Game Controller PCB v4 (Autodesk Fusion 360 design; units mm, degrees)
Autodesk Fusion 360 part; units mm, degrees
sketch "Sketch5" plane through (0, 0, 0) normal (0, 0, 1) x (1, 0, 0) in component "case"
  line L0 (-57.6, 75) -> (57.6, 75)
  line L1 (57.6, 75) -> (97.6, 5.718)
  line L2 (97.6, 5.718) -> (78.1684, -17.1384)
  line L3 (78.1684, -17.1384) -> (42.026, 0)
  line L4 (42.026, 0) -> (-42.026, 0)
  line L5 (-42.026, 0) -> (-78.1684, -17.1384)
  line L6 (-78.1684, -17.1384) -> (-97.6, 5.718)
  line L7 (-97.6, 5.718) -> (-57.6, 75)
  line L8 (0, 0) -> (0, 150) construction
  dimension "d31" = 57.6
  dimension "d32" = 80
  dimension "d34" = 80
  dimension "d35" = 120
  dimension "d36" = 120
  dimension "d37" = 30
  dimension "d38" = 40
  dimension "d39" = 30
  dimension "d40" = 40
  dimension "d41" = 105
  dimension "d42" = 105
  dimension "d43" = 75
  dimension "d44" = 57.6
  constraint horizontal L0
  constraint parallel L0 L4
  constraint midpoint L8.start L4
  constraint coincident L8.start origin
  constraint perpendicular L0 L8
  constraint midpoint L0 L8
  measures "d31" distance of L0.end L8
  measures "d32" distance of L0.start L6.end
  measures "d34" distance of L0.end L1.end
  measures "d35" angle of L0 L7
  measures "d36" angle of L0 L1
  measures "d37" distance of L1.end L2.end
  measures "d38" distance of L2.end L3.end
  measures "d39" distance of L5.end L6.end
  measures "d40" distance of L4.end L5.end
  measures "d41" angle of L2 L3
  measures "d42" angle of L5 L6
  measures "d43" distance of L0 L4
  measures "d44" distance of L0.start L8
extrude "Extrude1" add sketch "Sketch5" along normal blind 20 in component "case"
fillet "Fillet1" radius 10 8 edges at (42.026, 0, 10) (-42.026, 0, 10) (-78.1684, -17.1384, 10) (78.1684, -17.1384, 10) (97.6, 5.718, 10) (57.6, 75, 10) (-57.6, 75, 10) (-97.6, 5.718, 10) in component "case"
shell "Shell1" thickness 3 removed faces 1 at (-13.2584, 50, 20) in component "case"
sketch "Sketch7" plane through (0, 0, 3) normal (0, 0, 1) x (-1, 0, 0) in component "case"
  arc A0 (91.4768, -10.3237) -> (90.7478, -2.2897) centre (85.4146, -6.8237) ccw
  line L0 (90.7478, -2.2897) -> (80.8529, 9.3491)
  arc A1 (80.8529, 9.3491) -> (72.5205, 11.14) centre (75.5198, 4.8151) ccw
  line L1 (72.5205, 11.14) -> (45.3451, -1.7463)
  arc A2 (39.7752, -3) -> (45.3451, -1.7463) centre (39.7752, 10) ccw
  line L2 (39.7752, -3) -> (-39.7752, -3)
  arc A3 (-45.3451, -1.7463) -> (-39.7752, -3) centre (-39.7752, 10) ccw
  line L3 (-45.3451, -1.7463) -> (-72.5205, 11.14)
  arc A4 (-72.5205, 11.14) -> (-80.8529, 9.3491) centre (-75.5198, 4.8151) ccw
  line L4 (-80.8529, 9.3491) -> (-90.7478, -2.2897)
  arc A5 (-90.7478, -2.2897) -> (-91.4768, -10.3237) centre (-85.4146, -6.8237) ccw
  line L5 (-91.4768, -10.3237) -> (-57.8887, -68.5)
  arc A6 (-57.8887, -68.5) -> (-51.8265, -72) centre (-51.8265, -65) ccw
  line L6 (-51.8265, -72) -> (51.8265, -72)
  arc A7 (51.8265, -72) -> (57.8887, -68.5) centre (51.8265, -65) ccw
  line L7 (57.8887, -68.5) -> (91.4768, -10.3237)
  line L8 (56.1566, -67.5) -> (89.7447, -9.3237)
  arc A8 (89.7447, -9.3237) -> (89.224, -3.5851) centre (85.4146, -6.8237) ccw
  line L9 (89.224, -3.5851) -> (79.3291, 8.0537)
  arc A9 (79.3291, 8.0537) -> (73.3775, 9.3329) centre (75.5198, 4.8151) ccw
  line L10 (73.3775, 9.3329) -> (46.2021, -3.5534)
  arc A10 (39.7752, -5) -> (46.2021, -3.5534) centre (39.7752, 10) ccw
  line L11 (39.7752, -5) -> (-39.7752, -5)
  arc A11 (-46.2021, -3.5534) -> (-39.7752, -5) centre (-39.7752, 10) ccw
  line L12 (-46.2021, -3.5534) -> (-73.3775, 9.3329)
  arc A12 (-73.3775, 9.3329) -> (-79.3291, 8.0537) centre (-75.5198, 4.8151) ccw
  line L13 (-79.3291, 8.0537) -> (-89.224, -3.5851)
  arc A13 (-89.224, -3.5851) -> (-89.7447, -9.3237) centre (-85.4146, -6.8237) ccw
  line L14 (-89.7447, -9.3237) -> (-56.1566, -67.5)
  arc A14 (-56.1566, -67.5) -> (-51.8265, -70) centre (-51.8265, -65) ccw
  line L15 (-51.8265, -70) -> (51.8265, -70)
  arc A15 (51.8265, -70) -> (56.1566, -67.5) centre (51.8265, -65) ccw
  circle A16 centre (51.8265, -65) radius 1.5
  circle A17 centre (-51.8265, -65) radius 1.5
  circle A18 centre (-75.5198, 4.8151) radius 1.5
  circle A19 centre (-85.4146, -6.8237) radius 1.5
  circle A20 centre (75.5198, 4.8151) radius 1.5
  circle A21 centre (85.4146, -6.8237) radius 1.5
  dimension "d50" = -2
  dimension "d51" = 3
  dimension "d52" = 3
  dimension "d53" = 3
  dimension "d54" = 3
  dimension "d55" = 3
  dimension "d56" = 3
  constraint concentric A7 A16
  constraint concentric A6 A17
  constraint concentric A4 A18
  constraint concentric A5 A19
  constraint concentric A1 A20
  constraint concentric A0 A21
  measures "d51" diameter of A16
  measures "d52" diameter of A17
  measures "d53" diameter of A18
  measures "d54" diameter of A19
  measures "d55" diameter of A20
  measures "d56" diameter of A21
sketch "Sketch3" plane through (0, 0, 20) normal (0, 0, 1) x (-1, 0, 0)
  arc A0 (39.7752, -3) -> (45.3451, -1.7463) centre (39.7752, 10) ccw
  line L0 (45.3451, -1.7463) -> (72.5205, 11.14)
  arc A1 (80.8529, 9.3491) -> (72.5205, 11.14) centre (75.5198, 4.8151) ccw
  line L1 (80.8529, 9.3491) -> (90.7478, -2.2897)
  arc A2 (91.4768, -10.3237) -> (90.7478, -2.2897) centre (85.4146, -6.8237) ccw
  line L2 (91.4768, -10.3237) -> (57.8887, -68.5)
  arc A3 (51.8265, -72) -> (57.8887, -68.5) centre (51.8265, -65) ccw
  line L3 (51.8265, -72) -> (-51.8265, -72)
  arc A4 (-57.8887, -68.5) -> (-51.8265, -72) centre (-51.8265, -65) ccw
  line L4 (-57.8887, -68.5) -> (-91.4768, -10.3237)
  arc A5 (-90.7478, -2.2897) -> (-91.4768, -10.3237) centre (-85.4146, -6.8237) ccw
  line L5 (-90.7478, -2.2897) -> (-80.8529, 9.3491)
  arc A6 (-72.5205, 11.14) -> (-80.8529, 9.3491) centre (-75.5198, 4.8151) ccw
  line L6 (-72.5205, 11.14) -> (-45.3451, -1.7463)
  arc A7 (-45.3451, -1.7463) -> (-39.7752, -3) centre (-39.7752, 10) ccw
  line L7 (-39.7752, -3) -> (39.7752, -3)
  arc A8 (94.0749, -11.8237) -> (93.0334, -0.3465) centre (85.4146, -6.8237) ccw
  line L8 (93.0334, -0.3465) -> (83.1385, 11.2923)
  arc A9 (83.1385, 11.2923) -> (71.2352, 13.8507) centre (75.5198, 4.8151) ccw
  line L9 (71.2352, 13.8507) -> (44.0598, 0.9644)
  arc A10 (39.7752, 0) -> (44.0598, 0.9644) centre (39.7752, 10) ccw
  line L10 (39.7752, 0) -> (-39.7752, 0)
  arc A11 (-44.0598, 0.9644) -> (-39.7752, 0) centre (-39.7752, 10) ccw
  line L11 (-44.0598, 0.9644) -> (-71.2352, 13.8507)
  arc A12 (-71.2352, 13.8507) -> (-83.1385, 11.2923) centre (-75.5198, 4.8151) ccw
  line L12 (-83.1385, 11.2923) -> (-93.0334, -0.3465)
  arc A13 (-93.0334, -0.3465) -> (-94.0749, -11.8237) centre (-85.4146, -6.8237) ccw
  line L13 (-94.0749, -11.8237) -> (-60.4868, -70)
  arc A14 (-60.4868, -70) -> (-51.8265, -75) centre (-51.8265, -65) ccw
  line L14 (-51.8265, -75) -> (51.8265, -75)
  arc A15 (51.8265, -75) -> (60.4868, -70) centre (51.8265, -65) ccw
  line L15 (60.4868, -70) -> (94.0749, -11.8237)
component "Component" placed x (1, 0, 0) y (0, 1, 0) z (0, 0, 1) at (0, 0, 0)
component "case" placed x (1, 0, 0) y (0, 1, 0) z (0, 0, 1) at (0, 0, 0) in component "Component"
